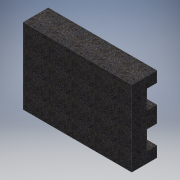
# Autodesk Inventor part: GraniteEpoxyBase
Saved by Autodesk Inventor 2016 (Build 200138000, 138)
## iProperties
Created: 2015-07-31
Part Number: GraniteEpoxyBase
Material: Concrete
Document SubType Name: Modeling
Designer: myhome
Density: 2.40731 g/cm^3
Appearance: Exposed Aggregate - Coarse
Mass: 388685 g
Surface Area: 28910 cm^2
Volume: 161460 cm^3
Author: myhome
Autodesk Inventor part; units mm, degrees
ref_plane "YZ Plane" through (0, 0, 0) normal (1, 0, 0) x (0, 1, 0)
ref_plane "XZ Plane" through (0, 0, 0) normal (0, 1, 0) x (-1, 0, 0)
ref_plane "XY Plane" through (0, 0, 0) normal (0, 0, 1) x (1, 0, 0)
sketch "Wireframe" plane through (0, 0, 0) normal (0, 0, 1) x (1, 0, 0)
  line L0 (0, 0) -> (1080, 0)
  line L1 (1080, 0) -> (1080, 750)
  line L2 (1080, 750) -> (0, 750)
  line L3 (0, 750) -> (0, 0)
  dimension "d0" = 1080
  dimension "d1" = 750
  constraints: 8 end point, 2 parallel, 1 horizontal, 1 perpendicular
  measures "d0" distance of L1.end L2.end
  measures "d1" distance of L0.end L1.end
extrude "Extrusion1" add sketch "Wireframe" along normal blind 250
sketch "Sketch4" plane through (1080, 0, 0) normal (1, 0, 0) x (0, 0, -1)
  line L0 (0, 0) -> (0, 750) projected
  line L1 (0, 0) -> (0, 149.657)
  line L2 (0, 0) -> (0, 105)
  line L3 (0, 0) -> (105, 0) construction
  line L4 (0, 105) -> (-100, 105)
  line L5 (-100, 105) -> (-100, 295)
  line L6 (-100, 295) -> (0, 295)
  line L7 (0, 295) -> (0, 455)
  line L8 (0, 455) -> (-100, 455)
  line L9 (-100, 455) -> (-100, 645)
  line L10 (-100, 645) -> (0, 645)
  line L11 (0, 645) -> (0, 750)
  dimension "d8" = 105
  dimension "d9" = 90
  dimension "d10" = 100
  dimension "d11" = 190
  dimension "d12" = 100
  dimension "d13" = 160
  dimension "d14" = 100
  dimension "d15" = 190
  dimension "d16" = 100
  constraints: 22 end point, 6 point on line, 3 perpendicular, 1 horizontal, 1 vertical
  measures "d8" distance of L0.start L2.end
  measures "d9" angle of L3 L2
  measures "d10" distance of L2.end L4.end
  measures "d11" distance of L4.end L5.end
  measures "d12" distance of L5.end L6.end
  measures "d13" distance of L6.end L7.end
  measures "d14" distance of L7.end L8.end
  measures "d15" distance of L8.end L9.end
  measures "d16" distance of L9.end L10.end
extrude "Extrusion2" cut sketch "Sketch4" against normal up to next contours L8 L9 L10 L0
sketch "Sketch5" plane through (1080, 0, 250) normal (1, 0, 0) x (0, 0, -1)
  line L0 (250, 0) -> (250, 105)
  line L1 (250, 0) -> (250, 455) projected
  line L2 (250, 105) -> (150, 105)
  line L3 (150, 105) -> (150, 295)
  line L4 (150, 295) -> (250, 295)
  dimension "d19" = 105
  dimension "d20" = 100
  dimension "d21" = 190
  dimension "d22" = 100
  constraints: 8 end point, 2 perpendicular, 2 point on line
  measures "d19" distance of L0.start L0.end
  measures "d20" distance of L0.end L2.end
  measures "d21" distance of L2.end L3.end
  measures "d22" distance of L3.end L4.end
extrude "Extrusion3" cut sketch "Sketch5" against normal up to next
body "Solid1"
